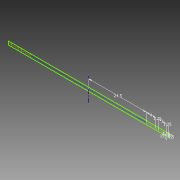
# Autodesk Inventor part: IDLER SHAFT
Saved by Autodesk Inventor 2014 (Build 180170000, 170)
## iProperties
Created: 2013-09-20
Part Number: IDLER SHAFT
Material: Generic
Document SubType Name: Modeling
Designer: Brandon
Density: 1 g/cm^3
Appearance: Default
Author: Brandon
Autodesk Inventor part; units mm, degrees
ref_plane "YZ Plane" through (0, 0, 0) normal (1, 0, 0) x (0, 1, 0)
ref_plane "XZ Plane" through (0, 0, 0) normal (0, 1, 0) x (-1, 0, 0)
ref_plane "XY Plane" through (0, 0, 0) normal (0, 0, 1) x (1, 0, 0)
sketch "Sketch1" plane through (0, 0, 0) normal (0, 1, 0) x (-1, 0, 0)
  line L0 (0, 0) -> (0, 5)
  line L1 (0, 0) -> (-24.5, 0) construction
  line L2 (-24.5, 0) -> (-28.5, 0) construction
  line L3 (-24.5, 0) -> (-20.5, 0) construction
  line L4 (-28.5, 0) -> (-29.75, 0) construction
  line L5 (-29.75, 0) -> (-32.75, 0) construction
  line L6 (-32.75, 0) -> (-34, 0) construction
  line L7 (-32.75, 0) -> (-32.8, 0) construction
  line L8 (-32.8, 0.65) -> (-32.9, 0.75)
  line L9 (-32.8, 0.65) -> (-32.7, 0.75)
  line L10 (-32.9, 0.75) -> (-34, 0.75)
  line L11 (-29.7, 0.65) -> (-29.6, 0.75)
  line L12 (-29.7, 0.65) -> (-29.8, 0.75)
  line L13 (-28.55, 0.65) -> (-28.65, 0.75)
  line L14 (-28.55, 0.65) -> (-28.45, 0.75)
  line L15 (-24.45, 0.65) -> (-24.35, 0.75)
  line L16 (-24.45, 0.65) -> (-24.55, 0.75)
  line L17 (0, 0) -> (24.5, 0) construction
  line L18 (24.5, 0) -> (28.5, 0) construction
  line L19 (24.5, 0) -> (20.5, 0) construction
  line L20 (28.5, 0) -> (29.75, 0) construction
  line L21 (29.75, 0) -> (32.75, 0) construction
  line L22 (32.75, 0) -> (34, 0) construction
  line L23 (32.75, 0) -> (32.8, 0) construction
  line L24 (32.8, 0.65) -> (32.9, 0.75)
  line L25 (32.8, 0.65) -> (32.7, 0.75)
  line L26 (32.9, 0.75) -> (34, 0.75)
  line L27 (29.7, 0.65) -> (29.6, 0.75)
  line L28 (29.7, 0.65) -> (29.8, 0.75)
  line L29 (28.55, 0.65) -> (28.65, 0.75)
  line L30 (28.55, 0.65) -> (28.45, 0.75)
  line L31 (24.45, 0.65) -> (24.55, 0.75)
  line L32 (24.45, 0.65) -> (24.35, 0.75)
  line L33 (-34, 0.75) -> (-34, 0)
  line L34 (34, 0.75) -> (34, 0)
  line L35 (29.8, 0.75) -> (32.7, 0.75)
  line L36 (28.65, 0.75) -> (29.6, 0.75)
  line L37 (0, 0.75) -> (24.35, 0.75)
  line L38 (24.55, 0.75) -> (28.45, 0.75)
  line L39 (0, 0.75) -> (-24.35, 0.75)
  line L40 (-24.55, 0.75) -> (-28.45, 0.75)
  line L41 (-28.65, 0.75) -> (-29.6, 0.75)
  line L42 (-29.8, 0.75) -> (-32.7, 0.75)
  line L43 (-34, 0) -> (34, 0)
  dimension "d5" = 24.5
  dimension "d7" = 4
  dimension "d9" = 1.25
  dimension "d11" = 3
  dimension "d13" = 1.25
  dimension "d17" = 0.05
  constraints: 88 end point, 6 horizontal, 5 perpendicular, 4 collinear, 2 parallel, 1 point on line
  measures "d5" distance of L0.start L1.end
  measures "d7" distance of L1.end L2.end
  measures "d9" distance of L2.end L4.end
  measures "d11" distance of L4.end L5.end
  measures "d13" distance of L5.end L6.end
  measures "d17" distance of L5.end L7.end
revolve "Revolution1" add sketch "Sketch1" angle 360 about axis through (0, 0, 0) along (1, 0, 0)
body "Solid1"
